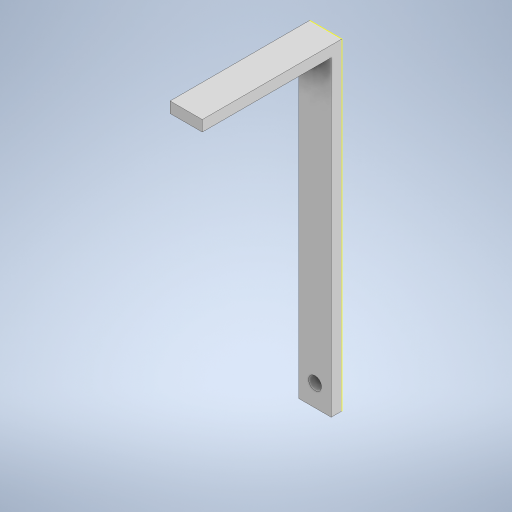
# Autodesk Inventor part: Part3
Saved by Autodesk Inventor 2023 (Build 270158000, 158)
## iProperties
Created: 2022-06-14
Part Number: Part3
Material: Generic
Document SubType Name: Modeling
Designer: care
Density: 1 g/cm^3
Appearance: Default
Author: care
Autodesk Inventor part; units mm, degrees
ref_plane "YZ Plane" through (0, 0, 0) normal (1, 0, 0) x (0, 1, 0)
ref_plane "XZ Plane" through (0, 0, 0) normal (0, 1, 0) x (-1, 0, 0)
ref_plane "XY Plane" through (0, 0, 0) normal (0, 0, 1) x (1, 0, 0)
sketch "Sketch1" plane through (0, 0, 0) normal (0, 1, 0) x (-1, 0, 0)
  point P0 (0, 0)
sketch "Sketch2" plane through (0, 0, 0) normal (0, 1, 0) x (-1, 0, 0)
  line L0 (3.1195, 2.6996) -> (-11.8805, 2.6996)
  line L1 (-11.8805, 2.6996) -> (-11.8805, -2.3004)
  line L2 (-11.8805, -2.3004) -> (3.1195, -2.3004)
  line L3 (3.1195, -2.3004) -> (3.1195, 2.6996)
  point P0 (0, 0)
  dimension "d0" = 15
  dimension "d1" = 5
  constraints: 8 end point, 2 parallel, 1 horizontal, 1 perpendicular
  measures "d0" distance of L2.end L1.end
  measures "d1" distance of L1.end L0.end
extrude "Extrusion1" add sketch "Sketch2" along normal blind 150
sketch "Sketch3" plane through (-3.1195, 0, 2.6996) normal (0, 0, 1) x (1, 0, 0)
  line L0 (15, 150) -> (0, 150) projected
  line L1 (15, 0) -> (15, 150) projected
  line L2 (0, 150) -> (15, 150)
  line L3 (15, 150) -> (15, 144.9614)
  line L4 (15, 144.9614) -> (0, 144.9614)
  line L5 (0, 144.9614) -> (0, 150)
  point P0 (3.1195, 0)
  constraints: 8 end point, 2 parallel, 1 horizontal, 1 perpendicular, 1 point on line
extrude "Extrusion2" add sketch "Sketch3" along normal blind 60
sketch "Sketch4" plane through (11.8805, 0, -2.3004) normal (0, 0, -1) x (-1, 0, 0)
  line L0 (0, 0) -> (15, 0) projected
  line L1 (0, 0) -> (15, 0) projected
  line L2 (15, 0) -> (15, 150) projected
  line L3 (0, 150) -> (15, 150) projected
  line L4 (0, 0) -> (0, 150) projected
  point P0 (11.8805, 0)
sketch "Sketch5" plane through (11.8805, 0, -2.3004) normal (0, 0, -1) x (-1, 0, 0)
  circle A0 centre (7.5, 10) radius 3 construction
  point P0 (11.8805, 0)
  dimension "d6" = 6
  constraints: 1 centre point, 1 coincident
  measures "d6" diameter of A0
hole "Hole1" at (4.3805, 10, -2.3004) direction (0, 0, 1) diameter 6 end through all
body "Solid1"
